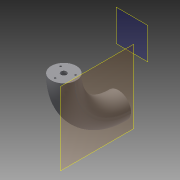
# Autodesk Inventor part: pole-corner
Saved by Autodesk Inventor 2014 (Build 180170000, 170)
## iProperties
Created: 2017-08-03
Part Number: pole-corner
Material: 一般
Document SubType Name: Modeling
Designer: hide
Density: 1 g/cm^3
Appearance: 既定
Author: hide
Autodesk Inventor part; units mm, degrees
ref_plane "XY Plane" through (0, 0, 0) normal (0, 0, 1) x (1, 0, 0)
sketch "スケッチ1" plane through (0, 0, 0) normal (0, 0, 1) x (1, 0, 0)
  circle A0 centre (0, 0) radius 17.5
  dimension "d0" = 35
  constraints: 1 centre point, 1 coincident
  measures "d0" diameter of A0
ref_plane "作業平面1" through (0, 95, 0) normal (0, 1, 0) x (-1, 0, 0)
sketch "スケッチ3" plane through (0, 0, 0) normal (1, 0, 0) x (0, 1, 0)
  arc A0 (0, 0) -> (75, -75) centre (75, 0) ccw
  dimension "d5" = 0
  dimension "d6" = 0
  dimension "d7" = 75
  constraints: 2 point on circle, 1 centre point
  measures "d5" vertical distance of A0.centre A0.start
  measures "d6" horizontal distance of A0.end A0.centre
  measures "d7" distance of A0.start A0.centre
sweep "スイープ1" add profiles "スケッチ1" path "スケッチ3"
sketch "スケッチ4" plane through (0, 0, 0) normal (0, 0, 1) x (1, 0, 0)
  circle A0 centre (0, 0) radius 17.5 projected
  circle A1 centre (0, 0) radius 4
  circle A2 centre (0, -12) radius 1.3
  circle A3 centre (10.3923, 6) radius 1.3
  circle A4 centre (-10.3923, 6) radius 1.3
  dimension "d9" = 8
  dimension "d10" = 2.6
  dimension "d11" = 12
  dimension "d12" = 0
  dimension "d15" = 360
  constraints: 4 centre point, 1 coincident, 7 other
  measures "d9" diameter of A1
  measures "d10" diameter of A2
  measures "d11" distance of A0.centre A2.centre
  measures "d12" horizontal distance of A2.centre A0.centre
extrude "押し出し1" cut sketch "スケッチ4" against normal blind 1.8 contours A1 | A2 | A3 | A4
shell "シェル1" thickness 1.5 removed faces 4 at (0.7574, 1.0973, -1.8) at (10.2386, 6.4052, -1.8) at (-10.0417, 6.3566, -1.8) at (-0.4801, -11.615, -1.8)
sketch "スケッチ5" plane through (0, 0, 0) normal (0, 0, 1) x (1, 0, 0)
  circle A0 centre (-10.3923, 6) radius 1.3 projected
  circle A1 centre (0, -12) radius 1.3 projected
  circle A2 centre (10.3923, 6) radius 1.3 projected
  circle A3 centre (-10.3923, 6) radius 2.8
  circle A4 centre (10.3923, 6) radius 2.8
  circle A5 centre (0, -12) radius 2.8
  dimension "d20" = 1.5
  dimension "d21" = 1.5
  dimension "d22" = 1.5
  constraints: 3 centre point, 3 coincident
  measures "d20" radial gap between concentric circles of A3 A0
  measures "d21" radial gap between concentric circles of A2 A4
  measures "d22" radial gap between concentric circles of A1 A5
extrude "押し出し2" add sketch "スケッチ5" against normal blind 6
sketch "スケッチ6" plane through (0, 75, -75) normal (0, 1, 0) x (1, 0, 0)
  circle A0 centre (0, 0) radius 17.5 projected
  circle A1 centre (0, 0) radius 2.5
  circle A2 centre (0, 12.5) radius 1.3
  circle A3 centre (-10.8253, -6.25) radius 1.3
  circle A4 centre (10.8253, -6.25) radius 1.3
  point P0 (0, -75)
  dimension "d26" = 5
  dimension "d27" = 2.6
  dimension "d28" = 12.5
  dimension "d31" = 360
  constraints: 4 centre point, 1 coincident, 7 other
  measures "d26" diameter of A1
  measures "d27" diameter of A2
  measures "d28" distance of A0.centre A2.centre
extrude "押し出し3" cut sketch "スケッチ6" against normal blind 3 contours A1 | A2 | A3 | A4
sketch "スケッチ7" plane through (0, 75, -75) normal (0, 1, 0) x (1, 0, 0)
  circle A0 centre (10.8253, -6.25) radius 1.3 projected
  circle A1 centre (0, 12.5) radius 1.3 projected
  circle A2 centre (-10.8253, -6.25) radius 1.3 projected
  circle A3 centre (0, 12.5) radius 2.8
  circle A4 centre (-10.8253, -6.25) radius 2.8
  circle A5 centre (10.8253, -6.25) radius 2.8
  point P0 (0, -75)
  dimension "d35" = 1.5
  dimension "d36" = 1.5
  dimension "d37" = 1.5
  constraints: 3 centre point, 3 coincident
  measures "d35" radial gap between concentric circles of A1 A3
  measures "d36" radial gap between concentric circles of A4 A2
  measures "d37" radial gap between concentric circles of A0 A5
extrude "押し出し4" add sketch "スケッチ7" against normal blind 6
fillet "フィレット2" radius 4 3 edges at (8.0253, 73.5, -68.75) (-13.6253, 73.5, -68.75) (-2.8, 73.5, -87.5)
ref_plane "作業平面2" through (17.4, 0, 0) normal (1, 0, 0) x (0, 1, 0)
sketch "スケッチ8" plane through (17.4, 0, 0) normal (1, 0, 0) x (0, 1, 0)
  line L0 (-41.6579, 27.2012) -> (94.8731, 27.2012)
  line L1 (94.8731, 27.2012) -> (94.8731, -100.1547)
  line L2 (94.8731, -100.1547) -> (-41.6579, -100.1547)
  line L3 (-41.6579, -100.1547) -> (-41.6579, 27.2012)
  point P0 (0, 0)
  constraints: 8 end point, 2 parallel, 1 horizontal, 1 perpendicular
extrude "押し出し5" cut sketch "スケッチ8" along normal blind 6
sketch "スケッチ9" plane through (0, 75, -75) normal (0, 1, 0) x (1, 0, 0)
  line L0 (17.4, -1.8682) -> (17.4, 1.8682) projected
  arc A0 (17.4, 1.8682) -> (17.4, -1.8682) centre (0, 0) ccw projected
  circle A1 centre (10.8253, -6.25) radius 1.3 projected
  circle A2 centre (0, 12.5) radius 1.3 projected
  circle A3 centre (-10.8253, -6.25) radius 1.3 projected
  circle A4 centre (0, 0) radius 2.5 projected
  point P0 (0, -75)
extrude "押し出し6" add sketch "スケッチ9" along normal blind 1
sketch "スケッチ10" plane through (0, 0, 0) normal (0, 0, 1) x (1, 0, 0)
  line L0 (17.4, -1.8682) -> (17.4, 1.8682) projected
  arc A0 (17.4, 1.8682) -> (17.4, -1.8682) centre (0, 0) ccw projected
  circle A1 centre (0, 0) radius 4 projected
  circle A2 centre (10.3923, 6) radius 1.3 projected
  circle A3 centre (-10.3923, 6) radius 1.3 projected
  circle A4 centre (0, -12) radius 1.3 projected
extrude "押し出し7" add sketch "スケッチ10" along normal blind 1
fillet "フィレット3" radius 4.5 3 edges at (-13.1923, 6, -1.5) (-2.8, -12, -1.5) (7.5923, 6, -1.5)
equation "\"d21\" = d20"
equation "\"d22\" = d20"
equation "\"d36\" = d35"
equation "\"d37\" = d36"
